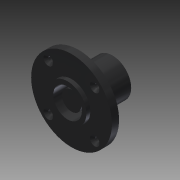
# Autodesk Inventor part: anschluss_strom
Saved by Autodesk Inventor 2015 (Build 190159000, 159)
## iProperties
Created: 2018-04-03
Part Number: anschluss_strom
Material: Generisch
Document SubType Name: Modeling
Designer: wepet
Density: 1 g/cm^3
Appearance: Vorgabe
Author: wepet
Autodesk Inventor part; units mm, degrees
ref_plane "YZ Plane" through (0, 0, 0) normal (1, 0, 0) x (0, 1, 0)
ref_plane "XZ Plane" through (0, 0, 0) normal (0, 1, 0) x (-1, 0, 0)
ref_plane "XY Plane" through (0, 0, 0) normal (0, 0, 1) x (1, 0, 0)
sketch "Skizze1" plane through (0, 0, 0) normal (0, 1, 0) x (-1, 0, 0)
  circle A0 centre (0, 0) radius 25.4
  dimension "d0" = 50.8
  constraints: 1 centre point, 1 coincident
  measures "d0" diameter of A0
extrude "Extrusion1" add sketch "Skizze1" along normal blind 4.5
sketch "Skizze2" plane through (0, 0, 0) normal (0, -1, 0) x (1, 0, 0)
  circle A0 centre (0, 0) radius 25.4 projected
  line L0 (-14.6, 14.6) -> (14.6, 14.6) construction
  line L1 (14.6, 14.6) -> (14.6, -14.6) construction
  line L2 (14.6, -14.6) -> (-14.6, -14.6) construction
  line L3 (-14.6, -14.6) -> (-14.6, 14.6) construction
  line L4 (0, 0) -> (14.6, 0) construction
  line L5 (0, 0) -> (0, 14.6) construction
  dimension "d3" = 29.2
  dimension "d4" = 29.2
  constraints: 12 end point, 4 coincident, 2 horizontal, 2 midpoint, 2 parallel, 1 perpendicular, 1 vertical
  measures "d3" distance of L0.start L0.end
  measures "d4" distance of L0.end L1.end
hole "Bohrung1" at (-14.6, 0, 14.6) at (14.6, 0, 14.6) at (14.6, 0, -14.6) at (-14.6, 0, -14.6) direction (0, 1, 0) diameter 3 end through all countersink diameter 6 countersink angle 90
sketch "Skizze3" plane through (0, 0, 0) normal (0, -1, 0) x (1, 0, 0)
  circle A0 centre (0, 0) radius 25.4 projected
  circle A1 centre (0, 0) radius 11.8
  dimension "d12" = 23.6
  constraints: 1 centre point, 1 coincident
  measures "d12" diameter of A1
extrude "Extrusion2" add sketch "Skizze3" along normal blind 2.5 contours A1
sketch "Skizze4" plane through (0, 4.5, 0) normal (0, 1, 0) x (1, 0, 0)
  circle A0 centre (0, 0) radius 25.4 projected
  circle A1 centre (0, 0) radius 25.4 projected
  circle A2 centre (0, 0) radius 11.8
  dimension "d15" = 23.6
  constraints: 1 centre point, 1 coincident
  measures "d15" diameter of A2
extrude "Extrusion3" add sketch "Skizze4" along normal blind 21.2 contours A2
sketch "Skizze5" plane through (0, -2.5, 0) normal (0, -1, 0) x (1, 0, 0)
  circle A0 centre (0, 0) radius 11.8 projected
  circle A1 centre (0, 0) radius 9
  circle A2 centre (0, 0) radius 6
  dimension "d18" = 18
  dimension "d19" = 12
  constraints: 2 centre point, 2 coincident
  measures "d18" diameter of A1
  measures "d19" diameter of A2
extrude "Extrusion4" cut sketch "Skizze5" against normal blind 15 contours A1
move faces "Verschieben1" translate (0, 2.5, 0) faces at (-0.7092, -2.5, 1.4219)
